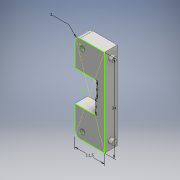
# Autodesk Inventor part: togh
Saved by Autodesk Inventor 2016 (Build 200138000, 138)
## iProperties
Created: 2017-05-26
Part Number: togh
Material: ABS Plastic
Document SubType Name: Modeling
Designer: Karol
Density: 1.06 g/cm^3
Appearance: Smooth - White
Author: Karol
Autodesk Inventor part; units mm, degrees
ref_plane "YZ Plane" through (0, 0, 0) normal (1, 0, 0) x (0, 1, 0)
ref_plane "XZ Plane" through (0, 0, 0) normal (0, 1, 0) x (-1, 0, 0)
ref_plane "XY Plane" through (0, 0, 0) normal (0, 0, 1) x (1, 0, 0)
sketch "Sketch1" plane through (0, 0, 0) normal (0, 1, 0) x (-1, 0, 0)
  line L0 (3.75, 17) -> (-5.75, 17)
  line L1 (-5.75, 17) -> (-5.75, -17)
  line L2 (-5.75, -17) -> (3.75, -17)
  line L3 (5.75, 17) -> (-5.75, -17) construction
  line L4 (-5.75, 17) -> (5.75, -17) construction
  arc A0 (5.75, 15) -> (3.75, 17) centre (3.75, 15) ccw
  arc A1 (3.75, -17) -> (5.75, -15) centre (3.75, -15) ccw
  line L5 (5.75, -15) -> (5.75, -6)
  line L6 (5.75, 6) -> (5.75, 15)
  line L7 (-2.25, 0) -> (-2.25, 6)
  line L8 (-2.25, 0) -> (-2.25, -6)
  line L9 (-2.25, -6) -> (5.75, -6)
  line L10 (5.75, 6) -> (-2.25, 6)
  point P0 (2.75, 14)
  point P1 (2.75, -14)
  point P2 (2.75, 0)
  dimension "d0" = 11.5
  dimension "d1" = 34
  dimension "d2" = 2
  dimension "d27" = 6
  dimension "d28" = 6
  constraints: 22 end point, 4 point on circle, 3 horizontal, 3 vertical, 2 centre point, 2 equal length, 2 point on line, 2 tangent, 1 equal radius, 1 perpendicular
  measures "d0" distance of L4.end L1.end
  measures "d1" distance of L1.end L0.end
  measures "d2" radius of A0
  measures "d27" distance of L7.start L7.end
  measures "d28" distance of L7.start L8.end
extrude "Extrusion1" add sketch "Sketch1" along normal blind 5
hole "Hole1" at (-2.75, 0, 14) at (-2.75, 0, -14) direction (0, 1, 0) diameter 1.778 depth 8 clearance for "Flat Head Machine Screw (82)" size "#0" standard "Ansi Unified Screw Threads"
sketch "Sketch2" plane through (5.75, 0, 17) normal (1, 0, 0) x (0, 0, -1)
  circle A0 centre (3, 2.5378) radius 1
  circle A1 centre (31, 2.5) radius 1
  point P0 (17, 0)
  dimension "d19" = 2
  dimension "d20" = 2
  dimension "d23" = 28
  constraints: 2 centre point, 2 coincident
  measures "d19" diameter of A0
  measures "d20" diameter of A1
  measures "d23" distance of A1.centre A0.centre
extrude "Extrusion2" add sketch "Sketch2" along normal blind 1.4
body "Solid1"
